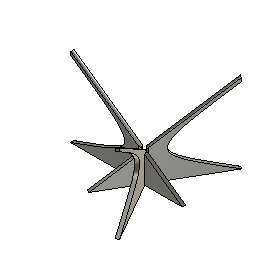
Cube Stand Interlock v1 (Autodesk Fusion 360 design; units mm, degrees)
Autodesk Fusion 360 part; units mm, degrees
note: some values were not read from the file. Chosen so that the rebuilt part matches the saved one: a side.
sketch "Sketch1" plane through (0, 0, 0) normal (0, 1, 0) x (1, 0, 0)
  line L0 (52.2558, 0) -> (-104.5116, -110.8513) construction
  line L1 (-104.5116, -110.8513) -> (-104.5116, 0) construction
  line L2 (-104.5116, 0) -> (52.2558, 0)
  line L3 (0, 0) -> (0, -36.9504) construction
  line L4 (0, -36.9504) -> (-104.5116, -36.9504) construction
  line L5 (0, -36.9504) -> (-104.5116, 0) construction
  line L6 (-25, -54.6281) -> (-25, -28.1116) construction
  spline S0 degree 5 poles (-104.5116, 0) (-97.2166, -2.5791) (-83.5843, -7.4484) (-66.0069, -13.8855) (-48.0515, -20.9174) (-33.4458, -28.1308) (-25.5247, -34.9872) (-23.4739, -42.6713) (-28.083, -51.9465) (-39.3938, -63.1802) (-56.4652, -76.5877) (-73.8658, -89.13) (-88.5876, -99.582) (-99.0891, -107.017) (-104.5116, -110.8513) knots 0 0 0 0 0 0 0.1 0.2 0.3 0.4 0.5 0.6 0.7 0.8 0.9 1 1 1 1 1 1
  line L7 (-80.3652, -93.7772) -> (-128.6579, -127.9253)
  line L8 (-139.7235, 12.4493) -> (-69.2996, -12.4493)
  line L9 (-25, -35.0869) -> (-25, -47.6528)
  line L10 (-104.5116, -110.8513) -> (-104.5116, -115.7502)
  line L11 (-104.5116, -115.7502) -> (59.184, 0)
  line L12 (59.184, 0) -> (52.2558, 0)
  point P0 (-25, -41.3698)
  dimension "d2" = 128
  dimension "d3" = 73.9008
  dimension "d4" = 52.2558
  dimension "d5" = 25
  dimension "d6" = 4
  constraint vertical L1
  constraint perpendicular L1 L2
  constraint coincident L3.start origin
  constraint coincident L0 L3.end
  constraint perpendicular L2 L3
  constraint coincident L1 L4.end
  constraint perpendicular L1 L4
  constraint coincident L3.start L2
  constraint coincident L0 L6.start
  constraint coincident L5 L6.end
  constraint perpendicular L4 L6
  constraint midpoint L6 P0
  constraint midpoint L0.end L7
  constraint coincident L0 L7.start
  constraint parallel L0 L7
  constraint midpoint L1.end L8
  constraint coincident L5 L8.end
  constraint parallel L5 L8
  constraint midpoint P0 L9
  constraint coincident L6 L9.start
  constraint parallel L1 L10
  constraint parallel L0 L11
  constraint collinear L2 L12
  measures "d2" distance of L0.end L3.end
  measures "d3" distance of L0.end L4.end
  measures "d4" distance of L3.start L0.start
  measures "d5" distance of L3.end L6
  measures "d6" distance of L0 L11
extrude "Extrude1" add sketch "Sketch1" along normal mid plane 5 makes body 1
ref_plane "WorkPlane1" through (-104.5116, 0, 115.7502) normal (-0.816497, 0, 0.57735) x (0, 1, 0)
sketch "Sketch2" plane through (-104.5116, 1.25, 115.7502) normal (-0.816497, 0, 0.57735) x (0, 1, 0)
  line L0 (-3.75, 0) -> (1.25, 0)
  line L1 (1.25, 0) -> (-1.25, -2.5) construction
  line L2 (1.25, 0) -> (3.8125, 0) construction
  line L3 (-1.25, -2.5) -> (-3.75, 0) construction
  arc A0 (1.25, 0) -> (-3.75, 0) centre (-1.25, -2.5) ccw
  dimension "d12" = 135
  dimension "d13" = 135
  constraint horizontal L2
  constraint coincident L0.end L1.start
  constraint coincident L0.start L3.end
  constraint coincident L1.end L3.start
  measures "d12" angle of L1 L2
  measures "d13" angle of L0 L3
extrude "Extrude2" cut sketch "Sketch2" against normal blind 128 bodies 1
pattern_circular "C-Pattern1" count 3 over 360 about axis through (0, 0, 1.75) along (0, 0, 1) of bodies 1 makes body 2 at (14.4805, -30.0809, 7.1941) makes body 3 at (18.8106, 27.5809, 7.1941)
sketch "Sketch4" plane through (0, 0, 0) normal (0, 1, 0) x (1, 0, 0)
  line L0 (0, 0) -> (0, -36.9504) construction
  line L1 (-104.5116, -115.7502) -> (59.184, 0) construction
  line L2 (-104.5116, 0) -> (52.2558, 0)
  line L3 (15, 0) -> (15, -65.0407)
  line L4 (-15, 0) -> (-15, -65.0407)
  line L5 (15, -14) -> (-15, -14)
  line L6 (15, -28) -> (-15, -28)
  line L7 (15, -58) -> (-15, -58)
  dimension "d24" = 15
  dimension "d25" = 14
  dimension "d26" = 14
  dimension "d27" = 30
  constraint coincident L2 L3.start
  constraint perpendicular L2 L3
  constraint symmetric L0 L3.start L4.start
  constraint symmetric L0 L3.end L4.end
  constraint coincident L3 L5.start
  constraint coincident L4 L5.end
  constraint perpendicular L4 L5
  constraint coincident L3 L6.start
  constraint coincident L4 L6.end
  constraint perpendicular L4 L6
  constraint coincident L3 L7.start
  constraint coincident L4 L7.end
  constraint perpendicular L4 L7
  measures "d24" distance of L0.start L3.start
  measures "d25" distance of L4.start L5.end
  measures "d26" distance of L5.end L6.end
  measures "d27" distance of L6.end L7.end
extrude "Extrude3" add sketch "Sketch4" along normal mid plane 5 separate body contours L2 L3 L4 L5 makes body 4
extrude "Extrude4" add sketch "Sketch4" along normal mid plane 5 separate body contours L3 L4 L5 L6 makes body 5
extrude "Extrude5" add sketch "Sketch4" along normal mid plane 5 separate body contours L3 L4 L6 L7 makes body 6
pattern_circular "C-Pattern2" count 3 over 360 about axis through (0, 0, 1.75) along (0, 0, 1) of bodies 4 makes body 7 at (0.3349, -5.5801, 4.6667) makes body 8 at (4.6651, 3.0801, 4.6667)
pattern_circular "C-Pattern3" count 3 over 360 about axis through (0, 0, 1.75) along (0, 0, 1) of bodies 5 makes body 9 at (-4.6651, 3.0801, 23.3333) makes body 10 at (-0.3349, -5.5801, 23.3333)
pattern_circular "C-Pattern4" count 3 over 360 about axis through (0, 0, 1.75) along (0, 0, 1) both ways of bodies 6 makes body 11 at (4.6651, 3.0801, 48) makes body 12 at (0.3349, -5.5801, 48)
combine "Combine5" operation cut target body 1 tool bodies 11 12 8 7 keep tools
combine "Combine6" operation cut target body 2 tool bodies 5 10 8 4 keep tools
combine "Combine7" operation cut target body 3 tool bodies 12 9 6 5 keep tools
delete_body "RemoveBody2" bodies 5
delete_body "RemoveBody3" bodies 12
delete_body "RemoveBody4" bodies 10
delete_body "RemoveBody5" bodies 9
delete_body "RemoveBody6" bodies 4
delete_body "RemoveBody7" bodies 6
delete_body "RemoveBody8" bodies 8
delete_body "RemoveBody9" bodies 7
delete_body "RemoveBody10" bodies 11
equation "side = 128 mm"
equation "d2 = side"
equation "d3 = side / sqrt(3)"
equation "d4 = side / sqrt(6)"
equation "d7 = plate_thickness / 2"
equation "d11 = -acos(sqrt(1 / 3))"
equation "d19 = -side"
equation "plate_thickness = 5 mm"
equation "d28 = plate_thickness / 2"
equation "d30 = plate_thickness / 2"
equation "d32 = plate_thickness / 2"
